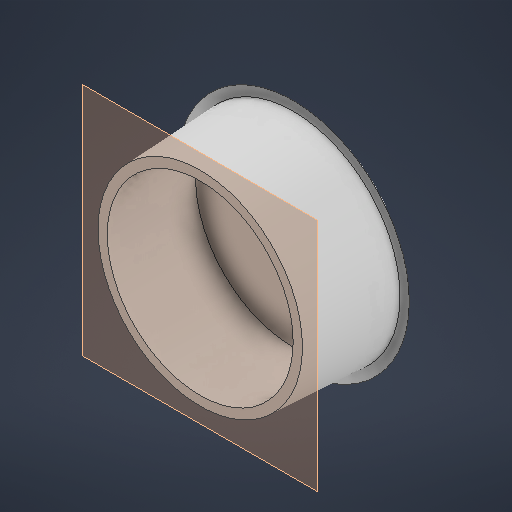
# Autodesk Inventor part: Стул ВВ
Saved by Autodesk Inventor 2025 (Build 290162000, 162)
## iProperties
Created: 2024-12-14
Part Number: Стул ВВ
Material: Типовые
Document SubType Name: Modeling
Designer: Phantom
Density: 1 g/cm^3
Appearance: По умолчанию
Author: Phantom
Autodesk Inventor part; units mm, degrees
ref_plane "YZ Plane" through (0, 0, 0) normal (1, 0, 0) x (0, 1, 0)
ref_plane "XZ Plane" through (0, 0, 0) normal (0, 1, 0) x (-1, 0, 0)
sketch "Эскиз1" plane through (0, 0, 0) normal (0, 0, 1) x (1, 0, 0)
  circle A0 centre (0, 0) radius 11.5
  circle A1 centre (0, 0) radius 10.5
  dimension "d0" = 23
  dimension "d7" = 21
  constraints: 2 centre point, 2 coincident
  measures "d0" diameter of A0
  measures "d7" diameter of A1
ref_plane "РабПлоскость1" through (0, 0, 10) normal (0, 0, 1) x (1, 0, 0)
sketch "Эскиз2" plane through (0, 0, 10) normal (0, 0, 1) x (1, 0, 0)
  circle A0 centre (0, 0) radius 11
  circle A1 centre (0, 0) radius 10
  dimension "d2" = 22
  dimension "d8" = 20
  constraints: 2 centre point, 2 coincident
  measures "d2" diameter of A0
  measures "d8" diameter of A1
loft "Лофт1" add profiles "Эскиз1", "Эскиз2" contours A0 | A1 / A0 | A1
sketch "Эскиз4" plane through (0, 0, 0) normal (0, 0, -1) x (-1, 0, 0)
  circle A0 centre (0, 0) radius 10.5
  circle A1 centre (0, 0) radius 11.5 projected
  dimension "d10" = 21
  constraints: 1 centre point, 1 coincident
  measures "d10" diameter of A0
sketch "Эскиз3" plane through (0, 0, 10) normal (0, 0, 1) x (1, 0, 0)
  circle A0 centre (0, 0) radius 10
  circle A1 centre (0, 0) radius 11 projected
  dimension "d9" = 20
  constraints: 1 centre point, 1 coincident
  measures "d9" diameter of A0
loft "Лофт2" cut profiles "Эскиз4", "Эскиз3" contours A0 / A0
sketch "Эскиз5" plane through (0, 0, 0) normal (0, 0, -1) x (-1, 0, 0)
  circle A0 centre (0, 0) radius 12.5
  dimension "d15" = 25
  constraints: 1 centre point, 1 coincident
  measures "d15" diameter of A0
extrude "Выдавливание1" add sketch "Эскиз5" along normal blind 2
fillet "Сопряжение1" radius 8 1 edges at (12.5, 0, -2)
